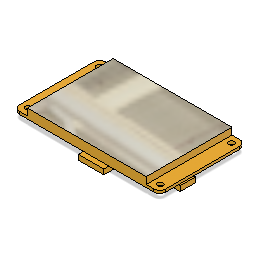
screen+EPS32+stand+v4 (Autodesk Fusion 360 archive; units mm, degrees)
design "ESP32-2432S028"
Autodesk Fusion 360 part; units mm, degrees
sketch "Sketch1" plane through (0, 0, 0) normal (0, 1, 0) x (1, 0, 0)
  line L0 (39.5, -25.25) -> (-39.5, -25.25)
  line L1 (-43, -21.75) -> (-43, 21.75)
  line L2 (-39.5, 25.25) -> (39.5, 25.25)
  line L3 (43, 21.75) -> (43, -21.75)
  line L4 (-43, -25.25) -> (43, 25.25) construction
  arc A0 (-39.5, 25.25) -> (-43, 21.75) centre (-39.5, 21.75) ccw
  arc A1 (-43, -21.75) -> (-39.5, -25.25) centre (-39.5, -21.75) ccw
  arc A2 (43, 21.75) -> (39.5, 25.25) centre (39.5, 21.75) ccw
  arc A3 (39.5, -25.25) -> (43, -21.75) centre (39.5, -21.75) ccw
  line L5 (39, -21) -> (-39, -21) construction
  line L6 (-39, -21) -> (-39, 21) construction
  line L7 (-39, 21) -> (39, 21) construction
  line L8 (39, 21) -> (39, -21) construction
  line L9 (39, -21) -> (-39, 21) construction
  line L10 (-39, -21) -> (39, 21) construction
  circle A4 centre (39, -21) radius 1.6
  circle A5 centre (39, 21) radius 1.6
  circle A6 centre (-39, 21) radius 1.6
  circle A7 centre (-39, -21) radius 1.6
  dimension "d3" = 3.5
  dimension "d4" = 78
  dimension "d5" = 42
  dimension "d6" = 3.2
  dimension "d7" = 3.2
  dimension "d8" = 3.2
  dimension "d9" = 3.2
  constraint horizontal L0
  constraint perpendicular L0 L1
  constraint parallel L0 L2
  constraint parallel L1 L3
  constraint coincident L4 origin
  constraint tangent L2 A0
  constraint tangent L1 A0
  constraint coincident L4.start L1
  constraint coincident L4.start L0
  constraint tangent L1 A1
  constraint tangent L0 A1
  constraint equal A0 A1
  constraint coincident L4.end L2
  constraint coincident L4.end L3
  constraint tangent L2 A2
  constraint tangent L3 A2
  constraint equal A0 A2
  constraint tangent L3 A3
  constraint tangent L0 A3
  constraint equal A0 A3
  constraint horizontal L5
  constraint perpendicular L5 L6
  constraint parallel L5 L7
  constraint parallel L6 L8
  constraint coincident L9 origin
  constraint coincident L10 origin
  constraint coincident L5.start L8.end
  constraint coincident L7.end L8.start
  constraint coincident L6.end L7.start
  constraint coincident L5.end L6.start
  measures "d3" radius of A0
  measures "d4" distance of L6.end L7.end
  measures "d5" distance of L5.end L6.end
  measures "d6" diameter of A4
  measures "d7" diameter of A5
  measures "d8" diameter of A6
  measures "d9" diameter of A7
extrude "Extrude1" add sketch "Sketch1" along normal blind 1.6
sketch "Sketch2" plane through (0, 1.6, 0) normal (0, 1, 0) x (-1, 0, 0)
  circle A0 centre (-39, -21) radius 1.6
  circle A1 centre (39, 21) radius 1.6
  circle A2 centre (-39, 21) radius 1.6
  circle A3 centre (39, -21) radius 1.6
  arc A4 (43, 21.75) -> (39.5, 25.25) centre (39.5, 21.75) ccw
  line L0 (39.5, 25.25) -> (-39.5, 25.25)
  arc A5 (-39.5, 25.25) -> (-43, 21.75) centre (-39.5, 21.75) ccw
  line L1 (-43, 21.75) -> (-43, -21.75)
  arc A6 (-43, -21.75) -> (-39.5, -25.25) centre (-39.5, -21.75) ccw
  line L2 (-39.5, -25.25) -> (39.5, -25.25)
  arc A7 (39.5, -25.25) -> (43, -21.75) centre (39.5, -21.75) ccw
  line L3 (43, -21.75) -> (43, 21.75)
  line L4 (43, -25.25) -> (35, -25.25)
  line L5 (-43, -25.25) -> (-35, -25.25)
  line L6 (-35, -25.25) -> (-35, 25.25)
  line L7 (35, -25.25) -> (35, 25.25)
  dimension "d12" = 8
  dimension "d13" = 8
  constraint perpendicular L3 L4
  constraint perpendicular L1 L5
  constraint coincident L0 L6.end
  constraint perpendicular L0 L6
  constraint coincident L0 L7.end
  constraint perpendicular L0 L7
  measures "d12" distance of L4.start L4.end
  measures "d13" distance of L5.start L5.end
extrude "Extrude2" add sketch "Sketch2" along normal blind 4 contours L0 L2 L6 L7
sketch "Sketch3" plane through (0, 0, 0) normal (0, -1, 0) x (1, 0, 0)
  circle A0 centre (39, -21) radius 1.6
  circle A1 centre (-39, 21) radius 1.6
  circle A2 centre (39, 21) radius 1.6
  circle A3 centre (-39, -21) radius 1.6
  arc A4 (-39.5, 25.25) -> (-43, 21.75) centre (-39.5, 21.75) ccw
  line L0 (-43, 21.75) -> (-43, -21.75)
  arc A5 (-43, -21.75) -> (-39.5, -25.25) centre (-39.5, -21.75) ccw
  line L1 (-39.5, -25.25) -> (39.5, -25.25)
  arc A6 (39.5, -25.25) -> (43, -21.75) centre (39.5, -21.75) ccw
  line L2 (43, -21.75) -> (43, 21.75)
  arc A7 (43, 21.75) -> (39.5, 25.25) centre (39.5, 21.75) ccw
  line L3 (39.5, 25.25) -> (-39.5, 25.25)
  line L4 (43, 25.25) -> (13, 25.25)
  line L5 (13, 25.25) -> (-2, 25.25)
  line L6 (-2, 25.25) -> (-2, 10.25)
  line L7 (-2, 10.25) -> (13, 10.25)
  line L8 (13, 10.25) -> (13, 25.25)
  line L9 (13, 25.25) -> (-2, 25.25)
  line L10 (-2, 25.25) -> (-2, 28.25)
  line L11 (-2, 28.25) -> (13, 28.25)
  line L12 (13, 28.25) -> (13, 25.25)
  line L13 (43, 25.25) -> (43, 14.25)
  line L14 (43, 14.25) -> (37, 14.25)
  line L15 (37, 14.25) -> (37, 5.25)
  line L16 (37, 5.25) -> (43, 5.25)
  line L17 (43, 5.25) -> (43, 14.25)
  line L18 (43, 14.25) -> (44, 14.25)
  line L19 (44, 14.25) -> (44, 5.25)
  line L20 (44, 5.25) -> (43, 5.25)
  line L21 (43, 5.25) -> (43, 14.25)
  dimension "d16" = 30
  dimension "d17" = 15
  dimension "d18" = 15
  dimension "d19" = 3
  dimension "d20" = 11
  dimension "d21" = 6
  dimension "d22" = 9
  dimension "d23" = 1
  dimension "d24" = 9
  constraint perpendicular L2 L4
  constraint horizontal L5
  constraint vertical L6
  constraint horizontal L7
  constraint vertical L8
  constraint horizontal L9
  constraint vertical L10
  constraint horizontal L11
  constraint vertical L12
  constraint perpendicular L4 L13
  constraint horizontal L14
  constraint vertical L15
  constraint horizontal L16
  constraint vertical L17
  constraint horizontal L18
  constraint vertical L19
  constraint horizontal L20
  constraint vertical L21
  measures "d16" distance of L4.start L4.end
  measures "d17" distance of L4.end L5.end
  measures "d18" distance of L4.end L7.end
  measures "d19" distance of L4.end L11.end
  measures "d20" distance of L4.start L13.end
  measures "d21" distance of L13.end L14.end
  measures "d22" distance of L13.end L16.end
  measures "d23" distance of L13.end L18.end
  measures "d24" distance of L13.end L16.end
extrude "Extrude3" add sketch "Sketch3" along normal blind 3 contours L3 L5 L9 L10 L11 L12 | L3 L5 L6 L7 L8 L9 | L2 L17 L18 L19 L20 L21 | L2 L14 L15 L16 L17 L21
